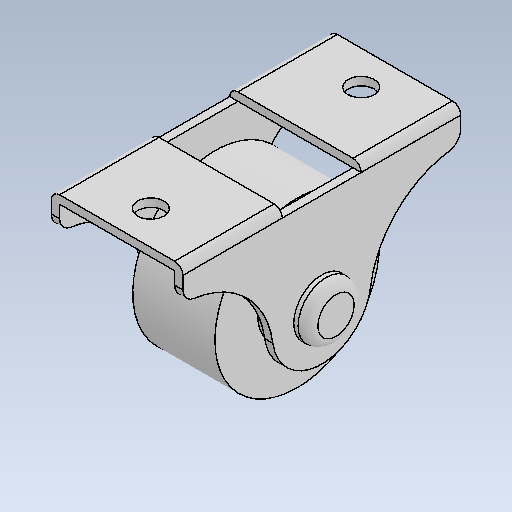
# Autodesk Inventor part: caster_d25
Saved by Autodesk Inventor 2026.2 (Build 302298010, 298A)
## iProperties
Created: 2026-03-19
Part Number: caster_d25
Material: Generic
Document SubType Name: Modeling
Designer: gakut
Density: 1 g/cm^3
Appearance: Default
Author: gakut
Autodesk Inventor part; units mm, degrees
ref_plane "YZ Plane" through (0, 0, 0) normal (1, 0, 0) x (0, 1, 0)
ref_plane "XZ Plane" through (0, 0, 0) normal (0, 1, 0) x (-1, 0, 0)
sketch "Sketch1" plane through (0, 0, 0) normal (1, 0, 0) x (0, 1, 0)
  circle A0 centre (0, 0) radius 12.5
  dimension "d0" = 25
  constraints: 1 centre point, 1 coincident
  measures "d0" diameter of A0
extrude "Extrusion1" add sketch "Sketch1" along normal blind 12.5
ref_plane "Work Plane1" through (6.25, 0, 0) normal (-1, 0, 0) x (0, 0, 1)
sketch "Sketch2" plane through (12.5, 0, 0) normal (1, 0, 0) x (0, 0, -1)
  circle A0 centre (0, 0) radius 6
  dimension "d3" = 12
  constraints: 1 centre point, 1 coincident
  measures "d3" diameter of A0
extrude "Extrusion2" add sketch "Sketch2" along normal blind 2.5
fillet "Fillet1" radius 2.5 1 edges at (15, 0, 6)
sketch "Sketch3" plane through (15, 0, 0) normal (1, 0, 0) x (0, 0, -1)
  circle A0 centre (0, 0) radius 7.5
  line L0 (-21.125, -11) -> (21.125, -11)
  line L1 (21.125, -11) -> (21.125, -16)
  line L2 (21.125, -16) -> (-21.125, -16)
  line L3 (-21.125, -16) -> (-21.125, -11)
  line L4 (-7.5, 0) -> (7.5, 0)
  line L5 (7.5, 0) -> (7.5, -11)
  line L6 (7.5, -11) -> (-7.5, -11)
  line L7 (-7.5, -11) -> (-7.5, 0)
  line L8 (6, -16) -> (-6, -16)
  line L9 (-6, -16) -> (-6, -14.75)
  line L10 (-6, -14.75) -> (6, -14.75)
  line L11 (6, -14.75) -> (6, -16)
  dimension "d7" = 15
  dimension "d8" = 16
  dimension "d9" = 5
  dimension "d10" = 42.25
  dimension "d11" = 21.125
  dimension "d21" = 12
  dimension "d22" = 6
  dimension "d23" = 1.25
  constraints: 24 end point, 6 parallel, 3 horizontal, 3 perpendicular, 2 point on circle, 2 point on line, 1 centre point, 1 coincident, 1 horizontal alignment, 1 midpoint
  measures "d7" diameter of A0
  measures "d8" distance from line of point (0, 0) L2
  measures "d9" distance of L0.end L1.end
  measures "d10" distance of L1.end L2.end
  measures "d11" distance from line of point (0, 0) L1
  measures "d21" distance of L9.end L10.end
  measures "d22" distance from line of point (0, 0) L9
  measures "d23" distance of L8.end L9.end
extrude "Extrusion3" add sketch "Sketch3" along normal blind 1.25 contours L4 A0 | L5 L0 L7 A0 | A0 L4 | L0 L1 L2 L11 L10 L9 L3
fillet "Fillet2" radius 14 2 edges at (15.625, -11, -7.5) (15.625, -11, 7.5)
fillet "Fillet3" radius 2 2 edges at (15.625, -10.999, 21.125) (15.625, -10.999, -21.125)
sketch "Sketch5" plane through (16.25, 0, 0) normal (1, 0, 0) x (0, 0, -1)
  circle A0 centre (0, 0) radius 4.265
  dimension "d25" = 8.53
  constraints: 1 centre point, 1 coincident
  measures "d25" diameter of A0
extrude "Extrusion5" add sketch "Sketch5" along normal blind 2.17
fillet "Fillet5" radius 1.5 1 edges at (18.42, 0, 4.265)
mirror "Mirror1" about plane through (6.25, 0, 0) normal (-1, 0, 0) of "Extrusion2", "Fillet1", "Extrusion3", "Fillet2", "Fillet3", "Extrusion5", "Fillet5"
sketch "Sketch4" plane through (-2.5, -16, 21.125) normal (1, 0, 0) x (0, 0, -1)
  line L0 (0, 0) -> (42.25, 0) projected
  line L1 (42.25, 0) -> (27.125, 0)
  line L2 (27.125, 0) -> (27.125, 1.25)
  line L3 (27.125, 1.25) -> (42.25, 1.25)
  line L4 (42.25, 1.25) -> (42.25, 0)
  line L5 (0, 0) -> (42.25, 0) projected
  line L6 (0, 0) -> (15.125, 0)
  line L7 (15.125, 0) -> (15.125, 1.25)
  line L8 (15.125, 1.25) -> (0, 1.25)
  line L9 (0, 1.25) -> (0, 0)
  point P0 (21.125, 16)
  point P1 (15.125, 0)
  point P2 (27.125, 0)
  point P3 (27.125, 1.25)
  point P4 (15.125, 1.25)
  dimension "d16" = 1.25
  constraints: 16 end point, 4 parallel, 2 coincident, 2 horizontal, 2 perpendicular, 1 point on line
  measures "d16" distance between parallel lines of L0 L8
extrude "Extrusion4" add sketch "Sketch4" along normal up to surface (17.5 mm away)
fillet "Fillet4" radius 1.25 4 edges at (-3.75, -16, -13.5625) (16.25, -16, -13.5625) (16.25, -16, 13.5625) (-3.75, -16, 13.5625)
sketch "Sketch6" plane through (-2.5, -16, 6) normal (0, -1, 0) x (1, 0, 0)
  line L0 (0, 15.125) -> (17.5, 15.125) projected
  point P0 (2.5, -6)
  point P1 (8.75, 10)
  point P2 (8.75, -22)
  point P3 (8.75, 15.125)
  dimension "d29" = 32
  dimension "d30" = 16
  constraints: 2 vertical alignment, 1 midpoint
  measures "d29" distance of point (8.75, 10) point (8.75, -22)
  measures "d30" vertical distance of point (2.5, -6) point (8.75, 10)
hole "Hole1" at (6.25, -16, 16) at (6.25, -16, -16) direction (0, 1, 0) diameter 4 end through all
equation "\"d11\" = 0.5 * d10"
equation "\"d22\" = 0.5 * d21"
equation "\"d30\" = 0.5 * d29"
body "Solid1"
